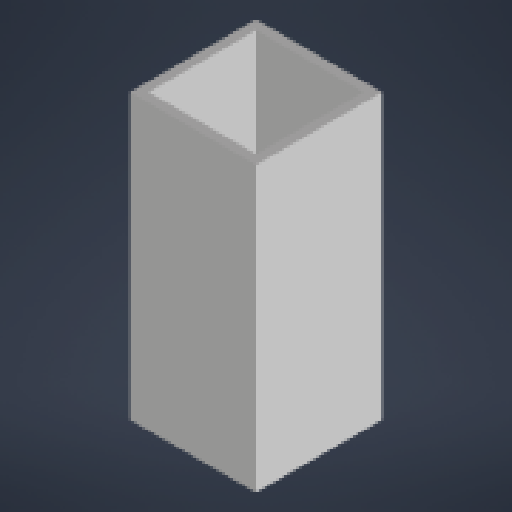
# Autodesk Inventor part: square_box_m_side_section
Saved by Autodesk Inventor 2024 (Build 280153000, 153)
## iProperties
Created: 2023-04-17
Part Number: square_box_m_side_section
Material: Типовые
Document SubType Name: Modeling
Designer: user
Density: 1 g/cm^3
Appearance: По умолчанию
Author: user
Autodesk Inventor part; units mm, degrees
ref_plane "YZ Plane" through (0, 0, 0) normal (1, 0, 0) x (0, 1, 0)
ref_plane "XZ Plane" through (0, 0, 0) normal (0, 1, 0) x (-1, 0, 0)
ref_plane "XY Plane" through (0, 0, 0) normal (0, 0, 1) x (1, 0, 0)
sketch "Эскиз1" plane through (0, 0, 0) normal (0, 0, 1) x (1, 0, 0)
  line L0 (0, 8) -> (1.5, 8) construction
  line L1 (0, 12) -> (1.5, 12) construction
  line L2 (0, -237) -> (0, 143) construction
  line L3 (20, -237) -> (20, 143) construction
  line L4 (0, 0) -> (20, 0)
  line L5 (20, 0) -> (20, 20)
  line L6 (20, 20) -> (0, 20)
  line L7 (0, 20) -> (0, 0)
  line L8 (1.5, 8) -> (1.5, 12) construction
  line L9 (1.5, 1.5) -> (18.5, 1.5)
  line L10 (18.5, 1.5) -> (18.5, 18.5)
  line L11 (18.5, 18.5) -> (1.5, 18.5)
  line L12 (1.5, 18.5) -> (1.5, 1.5)
  point P0 (0, 0)
  point P1 (1.5, 10)
  point P2 (0, 10)
  point P3 (18.5, 10)
  point P4 (10, 18.5)
  point P5 (10, 20)
  dimension "d0" = 20
  dimension "d1" = 1.5
  constraints: 22 end point, 5 midpoint, 4 horizontal, 4 parallel, 3 perpendicular, 2 horizontal alignment, 2 point on line, 1 vertical, 1 vertical alignment, 4 other
  measures "d0" distance of L6.end L4.start
  measures "d1" horizontal distance of point (0, 0) L9.start
ref_plane "РабПлоскость1" through (0, 123, 45) normal (0, 0, 1) x (1, 0, 0)
extrude "Выдавливание1" add sketch "Эскиз1" along normal up to surface (45 mm away)
sketch "Эскиз2" plane through (0, 0, 0) normal (-1, 0, 0) x (0, 0, 1)
  circle A0 centre (-6, 14) radius 2 construction
  circle A1 centre (-14, 6) radius 2 construction
  circle A2 centre (14, 137) radius 1.9999 construction
  circle A3 centre (6, 129) radius 1.65 construction
  circle A4 centre (14, 14) radius 2
  circle A5 centre (6, 6) radius 2
  point P0 (0, 0)
  constraints: 2 centre point, 2 equal radius, 2 horizontal alignment, 2 vertical alignment
extrude "Выдавливание2" cut sketch "Эскиз2" against normal through all
sketch "Эскиз3" plane through (0, 0, 0) normal (0, -1, 0) x (1, 0, 0)
  circle A0 centre (10, 37) radius 2 projected
  point P0 (0, 0)
extrude "Выдавливание3" cut sketch "Эскиз3" against normal through all
